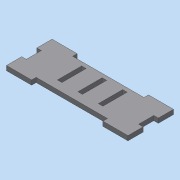
# Autodesk Inventor part: Camera-Holder_Bearing-Side
Saved by Autodesk Inventor 2016 SP1 (Build 200210100, 210)
## iProperties
Created: 2016-02-07
Part Number: Camera-Holder_Bearing-Side
Material: Generic
Document SubType Name: Modeling
Designer: Mohamed A.
Density: 1 g/cm^3
Appearance: Default
Author: Mohamed A.
Autodesk Inventor part; units mm, degrees
ref_plane "YZ Plane" through (0, 0, 0) normal (1, 0, 0) x (0, 1, 0)
ref_plane "XZ Plane" through (0, 0, 0) normal (0, 1, 0) x (-1, 0, 0)
ref_plane "XY Plane" through (0, 0, 0) normal (0, 0, 1) x (1, 0, 0)
sketch "Sketch1" plane through (0, 0, 0) normal (0, 0, 1) x (1, 0, 0)
  line L0 (-40, 15) -> (40, 15)
  line L1 (40, 15) -> (40, -15)
  line L2 (40, -15) -> (-40, -15)
  line L3 (-40, -15) -> (-40, 15)
  line L4 (-40, 15) -> (40, -15) construction
  line L5 (40, 15) -> (-40, -15) construction
  point P0 (0, 0)
  dimension "d0" = 80
  dimension "d1" = 30
  constraints: 12 end point, 2 midpoint, 2 parallel, 1 horizontal, 1 perpendicular
  measures "d0" distance of L1.end L2.end
  measures "d1" distance of L0.end L1.end
extrude "Extrusion1" add sketch "Sketch1" along normal mid plane 3
sketch "Sketch3" plane through (0, 0, 1.5) normal (0, 0, 1) x (1, 0, 0)
  line L0 (23.5315, 18) -> (23.5315, 15) projected
  line L1 (-23.4685, 18) -> (-23.4685, 15) projected
  line L2 (-23.4685, 15) -> (23.5315, 15)
  line L3 (23.5315, 15) -> (23.5315, 12)
  line L4 (23.5315, 12) -> (-23.4685, 12)
  line L5 (-23.4685, 12) -> (-23.4685, 15)
  line L6 (-40, 15) -> (-40, -15) projected
  line L7 (-40, 5) -> (-37, 5)
  line L8 (-37, 5) -> (-37, -5)
  line L9 (-37, -5) -> (-40, -5)
  line L10 (-40, -5) -> (-40, 5)
  line L11 (40, -15) -> (40, 15) projected
  line L12 (40, -5) -> (37, -5)
  line L13 (37, -5) -> (37, 5)
  line L14 (37, 5) -> (40, 5)
  line L15 (40, 5) -> (40, -5)
  line L16 (-40, -15) -> (40, -15) projected
  line L17 (40, 15) -> (-40, 15) projected
  line L18 (-23.4685, -15) -> (23.5315, -15)
  line L19 (23.5315, -15) -> (23.5315, -12)
  line L20 (23.5315, -12) -> (-23.4685, -12)
  line L21 (-23.4685, -12) -> (-23.4685, -15)
  line L22 (-14.9948, 8) -> (-11.9948, 8)
  line L23 (-11.9948, 8) -> (-11.9948, -8)
  line L24 (-11.9948, -8) -> (-14.9948, -8)
  line L25 (-14.9948, -8) -> (-14.9948, 8)
  line L26 (1.5, 8) -> (1.5, -8)
  line L27 (1.5, -8) -> (-1.5, -8)
  line L28 (-1.5, -8) -> (-1.5, 8)
  line L29 (-1.5, 8) -> (1.5, 8)
  line L30 (12.0052, 8) -> (15.0052, 8)
  line L31 (15.0052, 8) -> (15.0052, -8)
  line L32 (15.0052, -8) -> (12.0052, -8)
  line L33 (12.0052, -8) -> (12.0052, 8)
  dimension "d27" = 3
  dimension "d28" = 3
  dimension "d29" = 3
  dimension "d30" = 30
  dimension "d31" = 10
  dimension "d32" = 10
  dimension "d41" = 3
  constraints: 56 end point, 10 horizontal, 8 parallel, 6 vertical, 5 point on line, 4 collinear, 4 perpendicular, 12 other
  measures "d27" distance of L2.end L3.end
  measures "d28" distance of L8.end L9.end
  measures "d29" distance of L13.end L14.end
  measures "d30" distance between parallel lines of L16 L17
  measures "d31" distance between parallel lines of L17 L7
  measures "d32" distance between parallel lines of L16 L9
  measures "d41" distance of L19.end L18.end
extrude "Extrusion3" cut sketch "Sketch3" against normal blind 3 contours L2 L3 L4 L5 | L7 L8 L9 L6 | L11 L12 L13 L14 | L21 L20 L19 L16 | L22 L23 L24 L25 | L26 L27 L28 L29 | L30 L31 L32 L33
equation "\"d31\" = 0.333333 * d30"
equation "\"d32\" = d31"
body "Solid1"
